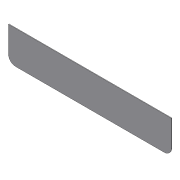
# Autodesk Inventor part: FE-00004-06
Saved by Autodesk Inventor 2012 (Build 160160000, 160)
## iProperties
Created: 2008-05-29
Part Number: FE-00004-06
Document SubType Name: Modeling
Designer: narosenberg
Density: 1 g/cm^3
Description: Shelf
Mass: 3941.66 g
Surface Area: 12678.2 cm^2
Volume: 3941.66 cm^3
Material: Default
Author: narosenberg
Autodesk Inventor part; units mm, degrees
ref_plane "YZ Plane" through (0, 0, 0) normal (1, 0, 0) x (0, 1, 0)
ref_plane "XZ Plane" through (0, 0, 0) normal (0, 1, 0) x (-1, 0, 0)
ref_plane "XY Plane" through (0, 0, 0) normal (0, 0, 1) x (1, 0, 0)
sketch "Sketch1" plane through (0, 0, 0) normal (0, 0, 1) x (1, 0, 0)
  line L0 (-36.8464, 19.8529) -> (1715.7536, 19.8529)
  line L1 (1715.7536, 19.8529) -> (1715.7536, -259.5471)
  line L2 (1639.5536, -335.7471) -> (39.3536, -335.7471)
  line L3 (-36.8464, -259.5471) -> (-36.8464, 19.8529)
  arc A0 (-36.8464, -259.5471) -> (39.3536, -335.7471) centre (39.3536, -259.5471) ccw
  arc A1 (1639.5536, -335.7471) -> (1715.7536, -259.5471) centre (1639.5536, -259.5471) ccw
  point P0 (-36.8464, -335.7471)
  dimension "d0" = 1752.6
  dimension "d1" = 355.6
  dimension "d2" = 76.2
  constraints: 8 end point, 4 point on circle, 4 tangent, 2 centre point, 2 parallel, 2 point on line, 1 equal radius, 1 horizontal, 1 perpendicular
  measures "d0" distance of L0.start L0.end
  measures "d1" distance of point (-36.846, -335.747) L0.start
  measures "d2" radius of A0
extrude "Extrusion1" add sketch "Sketch1" along normal blind 6.35
body "Solid1"
